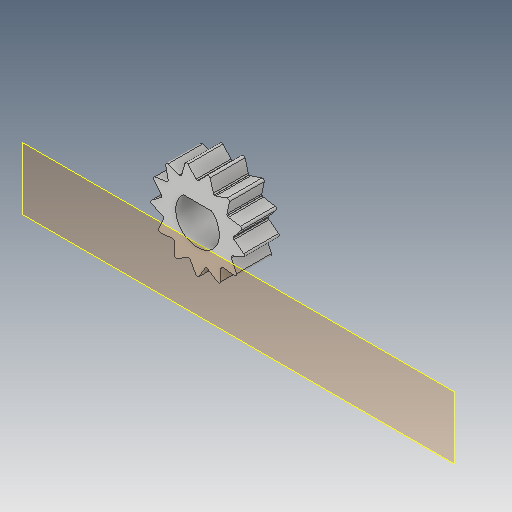
# Autodesk Inventor part: 00_gear_nema
Saved by Autodesk Inventor 2019.4 (Build 234330000, 330)
## iProperties
Created: 2021-02-14
Part Number: 00_gear_nema
Material: Generic
Document SubType Name: Modeling
Designer: diederichbenedict
Density: 1 g/cm^3
Appearance: Default
Author: diederichbenedict
Autodesk Inventor part; units mm, degrees
ref_plane "YZ Plane" through (0, 0, 0) normal (1, 0, 0) x (0, 1, 0)
ref_plane "XZ Plane" through (0, 0, 0) normal (0, 1, 0) x (-1, 0, 0)
ref_plane "XY Plane" through (0, 0, 0) normal (0, 0, 1) x (1, 0, 0)
ref_plane "Work Plane1" through (0, 0, 0) normal (0, 0, 1) x (1, 0, 0)
sketch "Sketch1" plane through (0, 0, 0) normal (0, 0, 1) x (1, 0, 0)
  line L0 (-22.5, -2) -> (22.5, -2) projected
  line L1 (22.5, -2) -> (22.5, 1) projected
  line L2 (22.5, 1) -> (21.2419, 1) projected
  line L3 (-20.9469, 1.1339) -> (-21.5112, 2.7464) projected
  line L4 (-22.5, 1) -> (-21.8888, 2.7464) projected
  line L5 (-22.5, 1) -> (-22.5, -2) projected
  circle A0 centre (-4.7, 6.94) radius 4.14
  circle A1 centre (-4.7, 6.94) radius 5.94 construction
  line L6 (-4.7, 1) -> (-12.3114, 1) construction
  line L7 (-4.7, 2.8) -> (-4.7, 1.5)
  line L8 (-4.7, 1.5) -> (-4.6, 1.5)
  line L9 (-4.6, 1.5) -> (-3.7978, 2.8995)
  arc A2 (20.4888, 2.7464) -> (20.1112, 2.7464) centre (20.3, 2.6803) ccw projected
  line L10 (19.5, 1) -> (20.1112, 2.7464) projected
  arc A3 (19.0531, 1.1339) -> (19.2419, 1) centre (19.2419, 1.2) ccw projected
  line L11 (19.0531, 1.1339) -> (18.4888, 2.7464) projected
  arc A4 (18.4888, 2.7464) -> (18.1112, 2.7464) centre (18.3, 2.6803) ccw projected
  line L12 (17.5, 1) -> (18.1112, 2.7464) projected
  arc A5 (17.0531, 1.1339) -> (17.2419, 1) centre (17.2419, 1.2) ccw projected
  line L13 (17.0531, 1.1339) -> (16.4888, 2.7464) projected
  arc A6 (16.4888, 2.7464) -> (16.1112, 2.7464) centre (16.3, 2.6803) ccw projected
  line L14 (15.5, 1) -> (16.1112, 2.7464) projected
  arc A7 (15.0531, 1.1339) -> (15.2419, 1) centre (15.2419, 1.2) ccw projected
  line L15 (15.0531, 1.1339) -> (14.4888, 2.7464) projected
  arc A8 (14.4888, 2.7464) -> (14.1112, 2.7464) centre (14.3, 2.6803) ccw projected
  line L16 (13.5, 1) -> (14.1112, 2.7464) projected
  arc A9 (13.0531, 1.1339) -> (13.2419, 1) centre (13.2419, 1.2) ccw projected
  line L17 (13.0531, 1.1339) -> (12.4888, 2.7464) projected
  arc A10 (12.4888, 2.7464) -> (12.1112, 2.7464) centre (12.3, 2.6803) ccw projected
  line L18 (11.5, 1) -> (12.1112, 2.7464) projected
  arc A11 (11.0531, 1.1339) -> (11.2419, 1) centre (11.2419, 1.2) ccw projected
  line L19 (11.0531, 1.1339) -> (10.4888, 2.7464) projected
  arc A12 (10.4888, 2.7464) -> (10.1112, 2.7464) centre (10.3, 2.6803) ccw projected
  line L20 (9.5, 1) -> (10.1112, 2.7464) projected
  arc A13 (9.0531, 1.1339) -> (9.2419, 1) centre (9.2419, 1.2) ccw projected
  line L21 (9.0531, 1.1339) -> (8.4888, 2.7464) projected
  arc A14 (8.4888, 2.7464) -> (8.1112, 2.7464) centre (8.3, 2.6803) ccw projected
  line L22 (7.5, 1) -> (8.1112, 2.7464) projected
  arc A15 (7.0531, 1.1339) -> (7.2419, 1) centre (7.2419, 1.2) ccw projected
  line L23 (7.0531, 1.1339) -> (6.4888, 2.7464) projected
  arc A16 (6.4888, 2.7464) -> (6.1112, 2.7464) centre (6.3, 2.6803) ccw projected
  line L24 (5.5, 1) -> (6.1112, 2.7464) projected
  arc A17 (5.0531, 1.1339) -> (5.2419, 1) centre (5.2419, 1.2) ccw projected
  line L25 (5.0531, 1.1339) -> (4.4888, 2.7464) projected
  arc A18 (4.4888, 2.7464) -> (4.1112, 2.7464) centre (4.3, 2.6803) ccw projected
  line L26 (3.5, 1) -> (4.1112, 2.7464) projected
  arc A19 (3.0531, 1.1339) -> (3.2419, 1) centre (3.2419, 1.2) ccw projected
  line L27 (3.0531, 1.1339) -> (2.4888, 2.7464) projected
  arc A20 (2.4888, 2.7464) -> (2.1112, 2.7464) centre (2.3, 2.6803) ccw projected
  line L28 (1.5, 1) -> (2.1112, 2.7464) projected
  arc A21 (1.0531, 1.1339) -> (1.2419, 1) centre (1.2419, 1.2) ccw projected
  line L29 (1.0531, 1.1339) -> (0.4888, 2.7464) projected
  arc A22 (0.4888, 2.7464) -> (0.1112, 2.7464) centre (0.3, 2.6803) ccw projected
  line L30 (-0.5, 1) -> (0.1112, 2.7464) projected
  arc A23 (-0.9469, 1.1339) -> (-0.7581, 1) centre (-0.7581, 1.2) ccw projected
  line L31 (-0.9469, 1.1339) -> (-1.5112, 2.7464) projected
  arc A24 (-1.5112, 2.7464) -> (-1.8888, 2.7464) centre (-1.7, 2.6803) ccw projected
  line L32 (-2.5, 1) -> (-1.8888, 2.7464) projected
  arc A25 (-2.9469, 1.1339) -> (-2.7581, 1) centre (-2.7581, 1.2) ccw projected
  line L33 (-2.9469, 1.1339) -> (-3.5112, 2.7464) projected
  arc A26 (-3.5112, 2.7464) -> (-3.8888, 2.7464) centre (-3.7, 2.6803) ccw projected
  line L34 (-4.5, 1) -> (-3.8888, 2.7464) projected
  arc A27 (-4.9469, 1.1339) -> (-4.7581, 1) centre (-4.7581, 1.2) ccw projected
  line L35 (-4.9469, 1.1339) -> (-5.5112, 2.7464) projected
  arc A28 (-5.5112, 2.7464) -> (-5.8888, 2.7464) centre (-5.7, 2.6803) ccw projected
  line L36 (-6.5, 1) -> (-5.8888, 2.7464) projected
  arc A29 (-6.9469, 1.1339) -> (-6.7581, 1) centre (-6.7581, 1.2) ccw projected
  line L37 (-6.9469, 1.1339) -> (-7.5112, 2.7464) projected
  arc A30 (-7.5112, 2.7464) -> (-7.8888, 2.7464) centre (-7.7, 2.6803) ccw projected
  line L38 (-8.5, 1) -> (-7.8888, 2.7464) projected
  arc A31 (-8.9469, 1.1339) -> (-8.7581, 1) centre (-8.7581, 1.2) ccw projected
  line L39 (-8.9469, 1.1339) -> (-9.5112, 2.7464) projected
  arc A32 (-9.5112, 2.7464) -> (-9.8888, 2.7464) centre (-9.7, 2.6803) ccw projected
  line L40 (-10.5, 1) -> (-9.8888, 2.7464) projected
  arc A33 (-10.9469, 1.1339) -> (-10.7581, 1) centre (-10.7581, 1.2) ccw projected
  line L41 (-10.9469, 1.1339) -> (-11.5112, 2.7464) projected
  arc A34 (-11.5112, 2.7464) -> (-11.8888, 2.7464) centre (-11.7, 2.6803) ccw projected
  line L42 (-12.5, 1) -> (-11.8888, 2.7464) projected
  arc A35 (-12.9469, 1.1339) -> (-12.7581, 1) centre (-12.7581, 1.2) ccw projected
  line L43 (-12.9469, 1.1339) -> (-13.5112, 2.7464) projected
  arc A36 (-13.5112, 2.7464) -> (-13.8888, 2.7464) centre (-13.7, 2.6803) ccw projected
  line L44 (-14.5, 1) -> (-13.8888, 2.7464) projected
  arc A37 (-14.9469, 1.1339) -> (-14.7581, 1) centre (-14.7581, 1.2) ccw projected
  line L45 (-14.9469, 1.1339) -> (-15.5112, 2.7464) projected
  arc A38 (-15.5112, 2.7464) -> (-15.8888, 2.7464) centre (-15.7, 2.6803) ccw projected
  line L46 (-16.5, 1) -> (-15.8888, 2.7464) projected
  arc A39 (-16.9469, 1.1339) -> (-16.7581, 1) centre (-16.7581, 1.2) ccw projected
  line L47 (-16.9469, 1.1339) -> (-17.5112, 2.7464) projected
  arc A40 (-17.5112, 2.7464) -> (-17.8888, 2.7464) centre (-17.7, 2.6803) ccw projected
  line L48 (-18.5, 1) -> (-17.8888, 2.7464) projected
  arc A41 (-18.9469, 1.1339) -> (-18.7581, 1) centre (-18.7581, 1.2) ccw projected
  line L49 (-18.9469, 1.1339) -> (-19.5112, 2.7464) projected
  arc A42 (-19.5112, 2.7464) -> (-19.8888, 2.7464) centre (-19.7, 2.6803) ccw projected
  line L50 (-20.5, 1) -> (-19.8888, 2.7464) projected
  arc A43 (-20.9469, 1.1339) -> (-20.7581, 1) centre (-20.7581, 1.2) ccw projected
  arc A44 (-21.5112, 2.7464) -> (-21.8888, 2.7464) centre (-21.7, 2.6803) ccw projected
  arc A45 (21.0531, 1.1339) -> (21.2419, 1) centre (21.2419, 1.2) ccw projected
  line L51 (21.0531, 1.1339) -> (20.4888, 2.7464) projected
  line L52 (19.5, 1) -> (19.2419, 1) projected
  line L53 (17.5, 1) -> (17.2419, 1) projected
  line L54 (15.5, 1) -> (15.2419, 1) projected
  line L55 (13.5, 1) -> (13.2419, 1) projected
  line L56 (11.5, 1) -> (11.2419, 1) projected
  line L57 (9.5, 1) -> (9.2419, 1) projected
  line L58 (7.5, 1) -> (7.2419, 1) projected
  line L59 (5.5, 1) -> (5.2419, 1) projected
  line L60 (3.5, 1) -> (3.2419, 1) projected
  line L61 (1.5, 1) -> (1.2419, 1) projected
  line L62 (-0.5, 1) -> (-0.7581, 1) projected
  line L63 (-2.5, 1) -> (-2.7581, 1) projected
  line L64 (-4.5, 1) -> (-4.7581, 1) projected
  line L65 (-6.5, 1) -> (-6.7581, 1) projected
  line L66 (-8.5, 1) -> (-8.7581, 1) projected
  line L67 (-10.5, 1) -> (-10.7581, 1) projected
  line L68 (-12.5, 1) -> (-12.7581, 1) projected
  line L69 (-14.5, 1) -> (-14.7581, 1) projected
  line L70 (-16.5, 1) -> (-16.7581, 1) projected
  line L71 (-18.5, 1) -> (-18.7581, 1) projected
  line L72 (-20.5, 1) -> (-20.7581, 1) projected
  point P0 (0, 0)
  dimension "d0" = 8.28
  dimension "d2" = 1.8
  dimension "d4" = 1.3
  dimension "d5" = 0.1
  dimension "d6" = 90
  dimension "d21" = 1
  dimension "d22" = 1
  dimension "d23" = 0
  constraints: 8 end point, 2 point on circle, 1 centre point, 1 horizontal, 1 perpendicular, 1 vertical alignment, 2 other
  measures "d0" diameter of A0
  measures "d4" distance of L7.start L7.end
  measures "d5" distance of L7.end L8.end
  measures "d6" angle of L8 L7
  measures "d21" horizontal distance of A28.centre A0.centre
  measures "d22" distance from line of A28.centre L7
  measures "d23" angle of L5 L7
extrude "Extrusion1" add sketch "Sketch1" against normal blind 4 contours L34 A26 L9 | L9 L8 L7 A0 A26 L34 | A0
mirror "Mirror1" about plane through (-4.7, 1.5, 0) normal (-1, 0, 0) of "Extrusion1"
fillet "Fillet1" radius 0.2 4 edges at (-5.6022, 2.8995, -2) (-3.7978, 2.8995, -2) (-4.6, 1.5, -2) (-4.8, 1.5, -2)
pattern_circular "Circular Pattern2" count 13 over 360 about axis through (-4.7, 6.94, 0) along (0, 0, -1) of "Extrusion1", "Mirror1", "Fillet1"
sketch "Sketch2" plane through (0, 0, 0) normal (0, 0, 1) x (1, 0, 0)
  arc A0 (-2.3851, 2.156) -> (-2.0779, 2.3173) centre (-2.2777, 2.3247) ccw projected
  line L0 (-2.0266, 3.6947) -> (-2.0779, 2.3173) projected
  arc A1 (-1.9592, 3.8372) -> (-2.0266, 3.6947) centre (-1.8268, 3.6873) ccw projected
  arc A2 (-1.9592, 3.8372) -> (-1.9502, 3.8452) centre (-4.7, 6.94) ccw projected
  arc A3 (-1.8006, 3.895) -> (-1.9502, 3.8452) centre (-1.8173, 3.6957) ccw projected
  line L1 (-1.8006, 3.895) -> (-0.4271, 3.7798) projected
  arc A4 (-0.4271, 3.7798) -> (-0.2299, 4.0654) centre (-0.4104, 3.9791) ccw projected
  line L2 (-0.8247, 5.3088) -> (-0.2299, 4.0654) projected
  arc A5 (-0.8312, 5.4663) -> (-0.8247, 5.3088) centre (-0.6443, 5.3951) ccw projected
  arc A6 (-0.8312, 5.4663) -> (-0.8269, 5.4776) centre (-4.7, 6.94) ccw projected
  arc A7 (-0.7176, 5.5912) -> (-0.8269, 5.4776) centre (-0.6398, 5.4069) ccw projected
  line L3 (-0.7176, 5.5912) -> (0.5521, 6.1275) projected
  arc A8 (0.5521, 6.1275) -> (0.5939, 6.472) centre (0.4743, 6.3117) ccw projected
  line L4 (-0.5105, 7.2966) -> (0.5939, 6.472) projected
  arc A9 (-0.5895, 7.433) -> (-0.5105, 7.2966) centre (-0.3909, 7.4569) ccw projected
  arc A10 (-0.5895, 7.433) -> (-0.5909, 7.445) centre (-4.7, 6.94) ccw projected
  arc A11 (-0.5469, 7.5964) -> (-0.5909, 7.445) centre (-0.3924, 7.4694) ccw projected
  line L5 (-0.5469, 7.5964) -> (0.3281, 8.6613) projected
  arc A12 (0.3281, 8.6613) -> (0.205, 8.9858) centre (0.1736, 8.7883) ccw projected
  line L6 (-1.1561, 9.2027) -> (0.205, 8.9858) projected
  arc A13 (-1.2894, 9.2868) -> (-1.1561, 9.2027) centre (-1.1247, 9.4002) ccw projected
  arc A14 (-1.2894, 9.2868) -> (-1.2963, 9.2967) centre (-4.7, 6.94) ccw projected
  arc A15 (-1.3277, 9.4512) -> (-1.2963, 9.2967) centre (-1.1318, 9.4106) ccw projected
  line L7 (-1.3277, 9.4512) -> (-1.0478, 10.8008) projected
  arc A16 (-1.0478, 10.8008) -> (-1.3075, 11.031) centre (-1.2436, 10.8415) ccw projected
  line L8 (-2.6136, 10.5904) -> (-1.3075, 11.031) projected
  arc A17 (-2.7707, 10.603) -> (-2.6136, 10.5904) centre (-2.6775, 10.7799) ccw projected
  arc A18 (-2.7707, 10.603) -> (-2.7814, 10.6086) centre (-4.7, 6.94) ccw projected
  arc A19 (-2.881, 10.7308) -> (-2.7814, 10.6086) centre (-2.6887, 10.7858) ccw projected
  line L9 (-2.881, 10.7308) -> (-3.2603, 12.0559) projected
  arc A20 (-3.2603, 12.0559) -> (-3.5973, 12.1389) centre (-3.4526, 12.0008) ccw projected
  line L10 (-4.549, 11.1419) -> (-3.5973, 12.1389) projected
  arc A21 (-4.694, 11.08) -> (-4.549, 11.1419) centre (-4.6937, 11.28) ccw projected
  arc A22 (-4.694, 11.08) -> (-4.706, 11.08) centre (-4.7, 6.94) ccw projected
  arc A23 (-4.851, 11.1419) -> (-4.706, 11.08) centre (-4.7063, 11.28) ccw projected
  line L11 (-4.851, 11.1419) -> (-5.8027, 12.1389) projected
  arc A24 (-5.8027, 12.1389) -> (-6.1397, 12.0559) centre (-5.9474, 12.0008) ccw projected
  line L12 (-6.519, 10.7308) -> (-6.1397, 12.0559) projected
  arc A25 (-6.6186, 10.6086) -> (-6.519, 10.7308) centre (-6.7113, 10.7858) ccw projected
  arc A26 (-6.6186, 10.6086) -> (-6.6293, 10.603) centre (-4.7, 6.94) ccw projected
  arc A27 (-6.7864, 10.5904) -> (-6.6293, 10.603) centre (-6.7225, 10.7799) ccw projected
  line L13 (-6.7864, 10.5904) -> (-8.0925, 11.031) projected
  arc A28 (-8.0925, 11.031) -> (-8.3522, 10.8008) centre (-8.1564, 10.8415) ccw projected
  line L14 (-8.0723, 9.4512) -> (-8.3522, 10.8008) projected
  arc A29 (-8.1037, 9.2967) -> (-8.0723, 9.4512) centre (-8.2682, 9.4106) ccw projected
  arc A30 (-8.1037, 9.2967) -> (-8.1106, 9.2868) centre (-4.7, 6.94) ccw projected
  arc A31 (-8.2439, 9.2027) -> (-8.1106, 9.2868) centre (-8.2753, 9.4002) ccw projected
  line L15 (-8.2439, 9.2027) -> (-9.605, 8.9858) projected
  arc A32 (-9.605, 8.9858) -> (-9.7281, 8.6613) centre (-9.5736, 8.7883) ccw projected
  line L16 (-8.8531, 7.5964) -> (-9.7281, 8.6613) projected
  arc A33 (-8.8091, 7.445) -> (-8.8531, 7.5964) centre (-9.0076, 7.4694) ccw projected
  arc A34 (-8.8091, 7.445) -> (-8.8105, 7.433) centre (-4.7, 6.94) ccw projected
  arc A35 (-8.8895, 7.2966) -> (-8.8105, 7.433) centre (-9.0091, 7.4569) ccw projected
  line L17 (-8.8895, 7.2966) -> (-9.9939, 6.472) projected
  arc A36 (-9.9939, 6.472) -> (-9.9521, 6.1275) centre (-9.8743, 6.3117) ccw projected
  line L18 (-8.6824, 5.5912) -> (-9.9521, 6.1275) projected
  arc A37 (-8.5731, 5.4776) -> (-8.6824, 5.5912) centre (-8.7602, 5.4069) ccw projected
  arc A38 (-8.5731, 5.4776) -> (-8.5688, 5.4663) centre (-4.7, 6.94) ccw projected
  arc A39 (-8.5753, 5.3088) -> (-8.5688, 5.4663) centre (-8.7557, 5.3951) ccw projected
  line L19 (-8.5753, 5.3088) -> (-9.1701, 4.0654) projected
  arc A40 (-9.1701, 4.0654) -> (-8.9729, 3.7798) centre (-8.9896, 3.9791) ccw projected
  line L20 (-7.5994, 3.895) -> (-8.9729, 3.7798) projected
  arc A41 (-7.4498, 3.8452) -> (-7.5994, 3.895) centre (-7.5827, 3.6957) ccw projected
  arc A42 (-7.4498, 3.8452) -> (-7.4408, 3.8372) centre (-4.7, 6.94) ccw projected
  arc A43 (-7.3734, 3.6947) -> (-7.4408, 3.8372) centre (-7.5732, 3.6873) ccw projected
  line L21 (-7.3734, 3.6947) -> (-7.3221, 2.3173) projected
  arc A44 (-7.3221, 2.3173) -> (-7.0149, 2.156) centre (-7.1223, 2.3247) ccw projected
  line L22 (-5.8522, 2.8963) -> (-7.0149, 2.156) projected
  arc A45 (-5.6966, 2.9217) -> (-5.8522, 2.8963) centre (-5.7448, 2.7276) ccw projected
  arc A46 (-5.6966, 2.9217) -> (-5.6849, 2.9189) centre (-4.7, 6.94) ccw projected
  arc A47 (-5.559, 2.8241) -> (-5.6849, 2.9189) centre (-5.7325, 2.7246) ccw projected
  line L23 (-5.559, 2.8241) -> (-4.8735, 1.6282) projected
  arc A48 (-4.8735, 1.6282) -> (-4.5265, 1.6282) centre (-4.7, 1.7277) ccw projected
  line L24 (-3.841, 2.8241) -> (-4.5265, 1.6282) projected
  arc A49 (-3.7151, 2.9189) -> (-3.841, 2.8241) centre (-3.6675, 2.7246) ccw projected
  arc A50 (-3.7151, 2.9189) -> (-3.7034, 2.9217) centre (-4.7, 6.94) ccw projected
  arc A51 (-3.5478, 2.8963) -> (-3.7034, 2.9217) centre (-3.6552, 2.7276) ccw projected
  line L25 (-3.5478, 2.8963) -> (-2.3851, 2.156) projected
  circle A52 centre (-4.7, 6.94) radius 2.5
  line L26 (-6.3021, 8.8592) -> (-3.0979, 8.8592)
  point P0 (0, 0)
  dimension "d24" = 5
  constraints: 2 end point, 2 point on circle, 1 centre point, 1 coincident, 1 horizontal
  measures "d24" diameter of A52
extrude "Extrusion2" cut sketch "Sketch2" against normal through all contours A52 L26 picked at (-4.9705, 7.1543)
body "Solid1"
